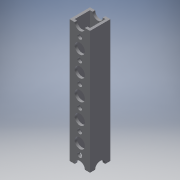
# Autodesk Inventor part: cube channel short
Saved by Autodesk Inventor 2016 (Build 200138000, 138)
## iProperties
Created: 2015-12-21
Part Number: cube channel short
Material: Generic
Document SubType Name: Modeling
Designer: tbloo
Density: 1 g/cm^3
Appearance: Default
Author: tbloo
Autodesk Inventor part; units mm, degrees
ref_plane "YZ Plane" through (0, 0, 0) normal (1, 0, 0) x (0, 1, 0)
ref_plane "XZ Plane" through (0, 0, 0) normal (0, 1, 0) x (-1, 0, 0)
ref_plane "XY Plane" through (0, 0, 0) normal (0, 0, 1) x (1, 0, 0)
sketch "Sketch1" plane through (0, 0, 0) normal (0, 0, 1) x (1, 0, 0)
  line L0 (8, -8) -> (-8, -8)
  line L1 (-8, -8) -> (-8, 8)
  line L2 (-8, 8) -> (8, 8)
  line L3 (8, 8) -> (8, -8)
  line L4 (8, -8) -> (-8, 8) construction
  line L5 (-8, -8) -> (8, 8) construction
  point P0 (0, 0)
  dimension "d0" = 16
  dimension "d1" = 16
  constraints: 12 end point, 2 midpoint, 2 parallel, 1 horizontal, 1 perpendicular
  measures "d0" distance of L1.end L2.end
  measures "d1" distance of L0.end L1.end
extrude "Extrusion1" add sketch "Sketch1" along normal blind 96
sketch "Sketch2" plane through (0, 0, 96) normal (0, 0, 1) x (1, 0, 0)
  line L0 (6, -6) -> (-6, -6)
  line L1 (-6, -6) -> (-6, 6)
  line L2 (-6, 6) -> (6, 6)
  line L3 (6, 6) -> (6, -6)
  line L4 (6, -6) -> (-6, 6) construction
  line L5 (-6, -6) -> (6, 6) construction
  point P0 (0, 0)
  dimension "d4" = 12
  dimension "d5" = 12
  constraints: 12 end point, 2 midpoint, 2 parallel, 1 horizontal, 1 perpendicular
  measures "d4" distance of L1.end L2.end
  measures "d5" distance of L0.end L1.end
extrude "Extrusion2" cut sketch "Sketch2" against normal blind 96
sketch "Sketch9" plane through (-8, -8, 0) normal (0, -1, 0) x (1, 0, 0)
  circle A0 centre (8, 0) radius 4
  dimension "d52" = 8
  constraints: 1 centre point, 1 coincident
  measures "d52" diameter of A0
hole "Hole7" at (0, -8, 0) direction (0, 1, 0) diameter 8 end through all
sketch "Sketch10" plane through (8, -8, 0) normal (1, 0, 0) x (0, 0, -1)
  circle A0 centre (0, 8) radius 4
  dimension "d60" = 8
  constraints: 1 centre point, 1 coincident
  measures "d60" diameter of A0
hole "Hole8" at (8, 0, 0) direction (-1, 0, 0) diameter 8 end through all
sketch "Sketch11" plane through (-8, -8, 96) normal (0, -1, 0) x (1, 0, 0)
  circle A0 centre (8, -88) radius 1.85 projected
  circle A1 centre (8, -72) radius 1.85 projected
  circle A2 centre (8, -56) radius 1.85 projected
  circle A3 centre (8, -40) radius 1.85 projected
  circle A4 centre (8, -24) radius 1.85 projected
  circle A5 centre (8, -8) radius 1.85 projected
  point P0 (8, -96)
hole "Hole9" at (0, -8, 8) at (0, -8, 24) at (0, -8, 40) at (0, -8, 56) at (0, -8, 72) at (0, -8, 88) direction (0, 1, 0) diameter 3.7 end through all
sketch "Sketch12" plane through (-8, -8, 96) normal (0, -1, 0) x (1, 0, 0)
  circle A0 centre (8, -80) radius 4 projected
  circle A1 centre (8, -64) radius 4 projected
  circle A2 centre (8, -48) radius 4 projected
  circle A3 centre (8, -32) radius 4 projected
  circle A4 centre (8, -16) radius 4 projected
  circle A5 centre (8, 0) radius 4 projected
  point P0 (8, -96)
hole "Hole10" at (0, -8, 16) at (0, -8, 32) at (0, -8, 48) at (0, -8, 64) at (0, -8, 80) at (0, -8, 96) direction (0, 1, 0) diameter 8 end through all
sketch "Sketch13" plane through (8, -8, 96) normal (1, 0, 0) x (0, 0, -1)
  circle A0 centre (88, 8) radius 1.85 projected
  circle A1 centre (72, 8) radius 1.85 projected
  circle A2 centre (56, 8) radius 1.85 projected
  circle A3 centre (40, 8) radius 1.85 projected
  circle A4 centre (24, 8) radius 1.85 projected
  circle A5 centre (8, 8) radius 1.85 projected
  point P0 (96, 8)
hole "Hole11" at (8, 0, 8) at (8, 0, 24) at (8, 0, 40) at (8, 0, 56) at (8, 0, 72) at (8, 0, 88) direction (-1, 0, 0) diameter 3.7 end through all
sketch "Sketch14" plane through (8, -8, 96) normal (1, 0, 0) x (0, 0, -1)
  circle A0 centre (80, 8) radius 4 projected
  circle A1 centre (64, 8) radius 4 projected
  circle A2 centre (48, 8) radius 4 projected
  circle A3 centre (32, 8) radius 4 projected
  circle A4 centre (16, 8) radius 4 projected
  circle A5 centre (0, 8) radius 4 projected
  point P0 (96, 8)
hole "Hole12" at (8, 0, 16) at (8, 0, 32) at (8, 0, 48) at (8, 0, 64) at (8, 0, 80) at (8, 0, 96) direction (-1, 0, 0) diameter 8 end through all
body "Solid1"
